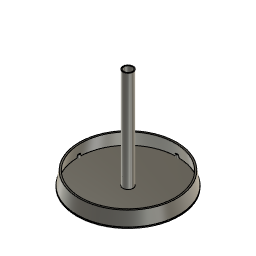
Custum Sculture Holder (Autodesk Fusion 360 design; units mm, degrees)
Autodesk Fusion 360 part; units mm, degrees
sketch "CircleSketch" plane through (0, 0, 0) normal (0, 0, 1) x (1, 0, 0)
  circle A0 centre (0, 0) radius 48.5
  circle A1 centre (0, 0) radius 50
  circle A2 centre (0, 0) radius 5
  circle A3 centre (0, 0) radius 4.1
  dimension "d6" = 100
  dimension "d7" = 10
  constraint coincident A0.centre A1.centre
  constraint concentric A0 A1
  constraint concentric A0 A2
  constraint concentric A2 A3
  measures "d6" diameter of A1
  measures "d7" diameter of A2
extrude "Extrude1" add sketch "CircleSketch" along normal blind 1.2 contours A0 | A1 | A2 | A3 makes body 1
extrude "Extrude2" add sketch "CircleSketch" along normal blind 10 contours A2 | A3 bodies 1
extrude "Extrude3" add sketch "CircleSketch" along normal blind 100 contours A2 bodies 1
sketch "Sketch2" plane through (0, 0, 0) normal (0, 1, 0) x (1, 0, 0)
extrude "Extrude4" add sketch "CircleSketch" along normal blind 13 separate body contours A1 makes body 2
sketch "Sketch3" plane through (0, 0, 0) normal (0, 0, 1) x (1, 0, 0)
  circle A0 centre (0, 0) radius 48.5
  line L0 (0, 0) -> (48.5, 0) construction
  line L1 (0, 0) -> (-48.5, 0) construction
  line L2 (0, 0) -> (0, 48.5) construction
  line L3 (0, 0) -> (0, -48.5) construction
  circle A1 centre (-48.5, 0) radius 1.5
  circle A2 centre (0, 48.5) radius 1.5
  circle A3 centre (0, 0) radius 50
  circle A4 centre (48.5, 0) radius 1.5
  circle A5 centre (0, -48.5) radius 1.5
  point P0 (-48.5, 0)
  point P1 (-50, 0)
  constraint coincident A0.centre L0.start
  constraint coincident A0 L0.end
  constraint coincident P0 L1.end
  constraint coincident A0 L2.end
  constraint perpendicular L0 L2
  constraint perpendicular L1 L2
  constraint coincident A0 L3.end
  constraint perpendicular L1 L3
  constraint coincident A1 P1
  constraint coincident L2.end A2.centre
  constraint tangent A2 A3
  constraint coincident L0.end A4.centre
  constraint tangent A3 A4
  constraint coincident L3.end A5.centre
  constraint tangent A3 A5
extrude "Extrude5" add sketch "Sketch3" along normal blind 4 separate body contours A0 A4 | A0 A4 | A0 A2 | A0 A2 | A0 A5 | A0 A5 | A0 A1 | A0 A1 makes body 3 at (-47.0019, -0.0748, 1.3333) makes body 4 at (0.4063, 47.0561, 2.6667) makes body 5 at (-1.4095, -49.013, 1.3333) makes body 6 at (49.9925, 0.1494, 2.6667)
move_body "Move1" bodies 2 to x (1, 0, 0) y (0, 1, 0) z (0, 0, 1) at (0, 0, 1)
combine "Combine1" operation add target body 5 tool bodies 2 3 4 6
draft "Draft1" angle -10 neutral plane through (0, 0, 1.2) pull (0, 0, 1) 1 faces at (6.5398, -48.0571, 6.3333) on bodies 5
draft "Draft2" angle 10 neutral plane through (0, 0, 1.2) pull (0, 0, 1) 1 faces at (-49.7627, 4.8656, 6.3333) on bodies 5
equation "Dimension = 100 mm"
equation "BorderSize = 3 mm"
equation "InnerDiameter = 10 mm"
equation "InnerBorder = 1.8 mm"
equation "d5 = ( Dimension - BorderSize )"
equation "d6 = Dimension"
equation "d7 = InnerDiameter"
equation "d8 = ( InnerDiameter - InnerBorder )"
equation "PlateHeight = 2 mm"
equation "PlateJoinHeight = 10 mm"
equation "TubeHeight = 100 mm"
equation "d14 = PlateJoinHeight"
equation "d16 = TubeHeight"
equation "d18 = HeightOfStuffHolder"
equation "d20 = PlateHeight + 2 mm"
equation "HeightOfStuffHolder = 13 mm"
